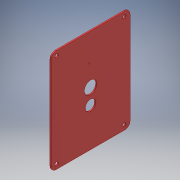
# Autodesk Inventor part: +XPanel_PCB
Saved by Autodesk Inventor 2018 (Build 220112000, 112)
## iProperties
Created: 2018-07-05
Part Number: +XPanel_PCB
Material: Epoxy Resin
Document SubType Name: Modeling
Designer: Bradley
Density: 1.14 g/cm^3
Appearance: Smooth - Red
Author: Bradley
Autodesk Inventor part; units mm, degrees
ref_plane "YZ Plane" through (0, 0, 0) normal (1, 0, 0) x (0, 1, 0)
ref_plane "XZ Plane" through (0, 0, 0) normal (0, 1, 0) x (-1, 0, 0)
ref_plane "XY Plane" through (0, 0, 0) normal (0, 0, 1) x (1, 0, 0)
sketch "Sketch1" plane through (0, 0, 0) normal (1, 0, 0) x (0, 1, 0)
  line L0 (-33, -49.5) -> (33, -49.5)
  line L1 (38, -44.5) -> (38, 44.5)
  line L2 (33, 49.5) -> (-33, 49.5)
  line L3 (-38, 44.5) -> (-38, -44.5)
  line L4 (-38, -49.5) -> (38, 49.5) construction
  line L5 (38, -49.5) -> (-38, 49.5) construction
  arc A0 (-33, 49.5) -> (-38, 44.5) centre (-33, 44.5) ccw
  arc A1 (38, 44.5) -> (33, 49.5) centre (33, 44.5) ccw
  arc A2 (33, -49.5) -> (38, -44.5) centre (33, -44.5) ccw
  arc A3 (-38, -44.5) -> (-33, -49.5) centre (-33, -44.5) ccw
  point P0 (0, 0)
  dimension "d0" = 76
  dimension "d1" = 99
  dimension "d2" = 5
  constraints: 12 end point, 8 point on circle, 8 point on line, 8 tangent, 4 centre point, 3 equal radius, 2 midpoint, 2 parallel, 1 horizontal, 1 perpendicular
  measures "d0" distance of L4.end L5.end
  measures "d1" distance of L5.end L4.start
  measures "d2" radius of A0
extrude "Extrusion1" add sketch "Sketch1" along normal mid plane 1
sketch "Sketch2" plane through (0.5, 0, 0) normal (1, 0, 0) x (0, 0, -1)
  line L0 (45, -32.5) -> (-45, -32.5) construction
  line L1 (-45, -32.5) -> (-45, 32.5) construction
  line L2 (-45, 32.5) -> (45, 32.5) construction
  line L3 (45, 32.5) -> (45, -32.5) construction
  line L4 (45, -32.5) -> (-45, 32.5) construction
  line L5 (-45, -32.5) -> (45, 32.5) construction
  point P0 (0, 0)
  dimension "d5" = 90
  dimension "d6" = 65
  constraints: 12 end point, 4 coincident, 2 midpoint, 2 parallel, 1 horizontal, 1 perpendicular
  measures "d5" distance of L1.end L2.end
  measures "d6" distance of L0.end L1.end
hole "Hole1" at (0.5, -32.5, 45) at (0.5, 32.5, 45) at (0.5, 32.5, -45) at (0.5, -32.5, -45) direction (-1, 0, 0) diameter 3.3 end through all
sketch "Sketch3" plane through (0.5, 0, 0) normal (1, 0, 0) x (0, 0, -1)
  circle A0 centre (-2.5, 0) radius 6
  circle A1 centre (12.35, 0) radius 5
  circle A2 centre (-23.25, -1.75) radius 0.475
  point P0 (0, 0)
  dimension "d14" = 14.85
  dimension "d15" = 12
  dimension "d16" = 10
  dimension "d19" = 2.5
  dimension "d20" = 23.25
  dimension "d21" = 1.75
  dimension "d22" = 0.95
  constraints: 3 centre point, 2 horizontal alignment, 1 coincident
  measures "d14" distance of A1.centre point (-2.5, 0)
  measures "d15" diameter of A0
  measures "d16" diameter of A1
  measures "d19" distance of point (0, 0) point (-2.5, 0)
  measures "d20" horizontal distance of point (0, 0) A2.centre
  measures "d21" vertical distance of point (0, 0) A2.centre
  measures "d22" diameter of A2
extrude "Extrusion2" cut sketch "Sketch3" against normal through all
body "Solid1"
